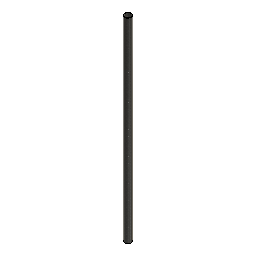
20021-012_small-tube (Autodesk Fusion 360 design; units mm, degrees)
Autodesk Fusion 360 part; units mm, degrees
sketch "Sketch1" plane through (0, 0, 0) normal (0, 0, 1) x (1, 0, 0)
  circle A0 centre (0, 0) radius 4.455
  circle A1 centre (0, 0) radius 5
  dimension "d2" = 10
  dimension "d6" = 8.91
  constraint coincident A0.centre A1.centre
  measures "d2" diameter of A1
  measures "d6" diameter of A0
extrude "Extrude1" add sketch "Sketch1" along normal blind 280
named bodies: "20021-005_arm"
